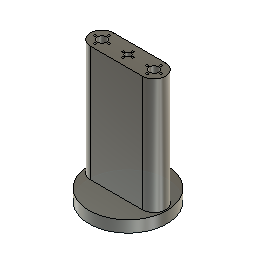
sls kolben 2 v5 (Autodesk Fusion 360 design; units mm, degrees)
Autodesk Fusion 360 part; units mm, degrees
sketch "Skizze1" plane through (0, 0, 0) normal (0, 0, 1) x (1, 0, 0)
  circle A0 centre (0, 0) radius 67.125
  dimension "d1" = 134.25
  constraint coincident A0.centre origin
  measures "d1" diameter of A0
extrude "Extrusion1" add sketch "Skizze1" along normal blind 10
extrude "Extrusion2" add 1 faces at (20.1592, 3.4821, 10) along direction (0, 0, 1) blind 10
sketch "Skizze2" plane through (0, 0, 20) normal (0, 0, 1) x (-1, 0, 0)
  circle A0 centre (0, 0) radius 67.125
  line L0 (0, 0) -> (-60, 0)
  line L1 (-60, 0) -> (-60, -10)
  line L2 (-60, -10) -> (0, -10)
  line L3 (0, -10) -> (0, 0)
  line L4 (-60, 0) -> (0, 0)
  line L5 (0, 0) -> (0, 10)
  line L6 (0, 10) -> (-60, 10)
  line L7 (-60, 10) -> (-60, 0)
  line L8 (0, -10) -> (60, -10)
  line L9 (60, -10) -> (60, 10)
  line L10 (60, 10) -> (0, 10)
  line L11 (0, 10) -> (0, -10)
  constraint horizontal L0
  constraint vertical L1
  constraint horizontal L2
  constraint vertical L3
  constraint coincident A0.centre L0.start
  constraint horizontal L4
  constraint vertical L5
  constraint horizontal L6
  constraint vertical L7
  constraint horizontal L8
  constraint vertical L9
  constraint horizontal L10
  constraint vertical L11
extrude "Extrusion3" add sketch "Skizze2" along normal blind 190 contours L0 L1 L2 L3 L4 L11 | L3 L5 L8 L9 L10 L11 | L0 L4 L5 L6 L7 L11
sketch "Skizze3" plane through (0, 0, 210) normal (0, 0, 1) x (-1, 0, 0)
  circle A0 centre (45, 0) radius 8
  circle A1 centre (-45, 0) radius 8
  dimension "d8" = 16
  dimension "d9" = 16
  measures "d8" diameter of A0
  measures "d9" diameter of A1
extrude "Extrusion4" add 1 faces at (-20, -10, 83.3333) along direction (0, -1, 0) blind 5
extrude "Extrusion5" add 1 faces at (20, 10, 83.3333) along direction (0, 1, 0) blind 5
sketch "Skizze4" plane through (0, 0, 210) normal (0, 0, 1) x (-1, 0, 0)
  circle A0 centre (0, 0) radius 5.25
  line L0 (0, 0) -> (-8, 0)
  line L1 (-8, 0) -> (0, 0)
  line L2 (0, 0) -> (8, 0)
  line L3 (0, 0) -> (0, 8)
  line L4 (0, 8) -> (0, -8)
  circle A1 centre (0, -8) radius 2
  circle A2 centre (8, 0) radius 2
  circle A3 centre (0, 8) radius 2
  circle A4 centre (-8, 0) radius 2
  line L5 (45, 0) -> (45, -12)
  line L6 (45, 0) -> (45, 12)
  line L7 (45, 12) -> (45, 0)
  line L8 (45, 0) -> (33, 0)
  line L9 (45, 0) -> (57, 0)
  line L10 (-45, 0) -> (-33, 0)
  line L11 (-33, 0) -> (-57, 0)
  line L12 (-45, 0) -> (-45, -12)
  line L13 (-45, -12) -> (-45, 12)
  circle A5 centre (-45, 0) radius 22.2036
  circle A6 centre (45, 0) radius 22.0227
  circle A7 centre (0, 0) radius 15
  circle A8 centre (-45, 12) radius 2
  circle A9 centre (-33, 0) radius 2
  circle A10 centre (-45, -12) radius 2
  circle A11 centre (-57, 0) radius 2
  circle A12 centre (45, -12) radius 2
  circle A13 centre (57, 0) radius 2
  circle A14 centre (45, 12) radius 2
  circle A15 centre (33, 0) radius 2
  dimension "d14" = 10.5
  dimension "d15" = 4
  dimension "d16" = 4
  dimension "d17" = 4
  dimension "d18" = 4
  dimension "d19" = 30
  dimension "d20" = 4
  dimension "d21" = 4
  dimension "d22" = 4
  dimension "d23" = 4
  dimension "d24" = 4
  dimension "d25" = 4
  dimension "d26" = 4
  dimension "d27" = 4
  constraint coincident A0.centre L0.start
  constraint horizontal L0
  constraint parallel L0 L2
  constraint perpendicular L2 L3
  constraint perpendicular L1 L4
  constraint coincident L4.end A1.centre
  constraint coincident L2.end A2.centre
  constraint coincident L3.end L4.start
  constraint coincident L0.end L1.start
  constraint vertical L5
  constraint parallel L5 L6
  constraint perpendicular L5 L8
  constraint perpendicular L7 L9
  constraint parallel L8 L10
  constraint parallel L10 L11
  constraint perpendicular L11 L12
  constraint perpendicular L11 L13
  constraint coincident L10.start L12.start
  constraint coincident L5.start L6.start
  constraint coincident L13.end A8.centre
  constraint coincident L10.end L11.start
  constraint coincident L12.end L13.start
  constraint coincident L11.end A11.centre
  constraint coincident L5.end A12.centre
  constraint coincident L9.end A13.centre
  constraint coincident L6.end L7.start
  constraint coincident L8.end A15.centre
  measures "d14" diameter of A0
  measures "d15" diameter of A1
  measures "d16" diameter of A2
  measures "d17" diameter of A3
  measures "d18" diameter of A4
  measures "d19" diameter of A7
  measures "d20" diameter of A8
  measures "d21" diameter of A9
  measures "d22" diameter of A10
  measures "d23" diameter of A11
  measures "d24" diameter of A12
  measures "d25" diameter of A13
  measures "d26" diameter of A14
  measures "d27" diameter of A15
extrude "Extrusion6" cut 1 faces at (-20, -15, 83.3333) along direction (0, 1, 0) blind 30
extrude "Extrusion7" add sketch "Skizze4" sketch "Skizze3" against normal blind 190 of sketch 2 contours A0
sketch "Skizze5" plane through (0, 0, 210) normal (0, 0, 1) x (-1, 0, 0)
  circle A0 centre (45, 12) radius 2
  circle A1 centre (57, 0) radius 2
  circle A2 centre (45, -12) radius 2
  circle A3 centre (33, 0) radius 2
  circle A4 centre (45, 0) radius 22.0227
  circle A5 centre (45, 0) radius 8
  circle A6 centre (-45, 0) radius 8
  dimension "d32" = 16
  dimension "d33" = 16
  constraint concentric A4 A5
  measures "d32" diameter of A5
  measures "d33" diameter of A6
extrude "Extrusion8" cut sketch "Skizze5" against normal blind 190 contours A5 | A6
extrude "Extrusion9" add 12 faces at (33.7124, 0.5212, 20) (43.8521, -11.4472, 20) (43.8521, 12.5528, 20) (57.8076, 0.4919, 20) (-0.1483, 8.5047, 20) (7.5843, -0.7199, 20) (0.4887, -7.5466, 20) (-7.4749, -0.0323, 20) (-34.1479, -0.5528, 20) (-43.614, -12.2526, 20) (-56.1924, 0.4919, 20) (-43.614, 11.7474, 20) along direction (0, 0, 1) blind 180
extrude "Extrusion10" add 3 faces at (38.0561, -11.8714, 210) (-7.5649, 5.256, 210) (-51.9063, -11.8242, 210) along direction (0, 0, 1) blind 10
extrude "Extrusion11" add 12 faces at (-56.1924, 0.4919, 200) (-43.614, 11.7474, 200) (-34.1479, -0.5528, 200) (-43.614, -12.2526, 200) (-0.1483, 8.5047, 200) (7.5843, -0.7199, 200) (0.4887, -7.5466, 200) (-7.4749, -0.0323, 200) (57.8076, 0.4919, 200) (43.8521, 12.5528, 200) (33.7124, 0.5212, 200) (43.8521, -11.4472, 200) along direction (0, 0, 1) blind 5
sketch "Skizze6" plane through (0, 0, 220) normal (0, 0, 1) x (-1, 0, 0)
  circle A0 centre (-45, 0) radius 8
  circle A1 centre (-33, 0) radius 2
  circle A2 centre (-57, 0) radius 2
  circle A3 centre (-45, -12) radius 2
  circle A4 centre (-45, 12) radius 2
  circle A5 centre (-45, 0) radius 22.2036
  circle A6 centre (45, 0) radius 20
  circle A7 centre (-45, 0) radius 20
  circle A8 centre (45, 0) radius 22.1359
  dimension "d42" = 40
  dimension "d43" = 40
  constraint concentric A5 A7
  constraint concentric A6 A8
  measures "d42" diameter of A6
  measures "d43" diameter of A7
extrude "Extrusion12" cut sketch "Skizze6" against normal blind 200 contours A5 | A8
sketch "Skizze7" plane through (0, 0, 0) normal (0, 0, -1) x (1, 0, 0)
  circle A0 centre (0, 0) radius 67.125
sketch "Skizze8" plane through (0, 0, 20) normal (0, 0, 1) x (-1, 0, 0)
  circle A0 centre (-45, 0) radius 20
  circle A1 centre (45, 0) radius 20
  circle A2 centre (0, 0) radius 67.125
  circle A3 centre (0, 0) radius 15
  line L0 (45, 20) -> (-45, 20)
  line L1 (-45, -20) -> (45, -20)
  constraint coincident A1 L0.start
  constraint coincident A0 L0.end
  constraint tangent A0 L0
  constraint coincident A0 L1.start
  constraint coincident A1 L1.end
  constraint tangent A1 L1
extrude "Extrusion13" add sketch "Skizze8" along normal up to surface (200 mm away) contours A0 A1 L0 L1
